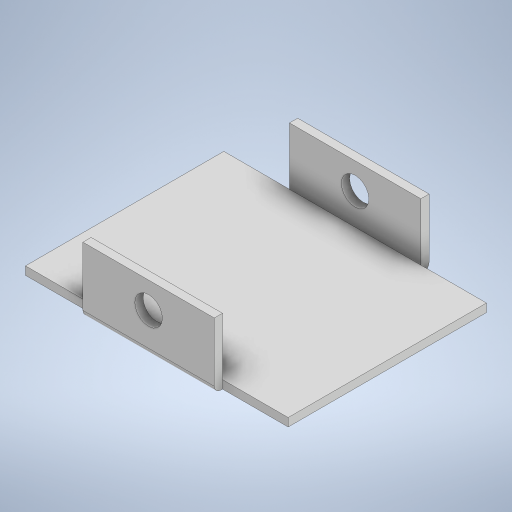
# Autodesk Inventor part: L1 Gearbox Cover Top
Saved by Autodesk Inventor 2024 (Build 280153000, 153)
## iProperties
Created: 2023-09-27
Part Number: L1 Gearbox Cover Top
Material: Generic
Document SubType Name: Modeling
Designer: lando
Density: 1 g/cm^3
Appearance: Default
Author: lando
Autodesk Inventor part; units mm, degrees
ref_plane "YZ Plane" through (0, 0, 0) normal (1, 0, 0) x (0, 1, 0)
ref_plane "XZ Plane" through (0, 0, 0) normal (0, 1, 0) x (-1, 0, 0)
ref_plane "XY Plane" through (0, 0, 0) normal (0, 0, 1) x (1, 0, 0)
sketch "Sketch1" plane through (0, 0, 0) normal (0, 1, 0) x (-1, 0, 0)
  line L0 (0, 0) -> (50.8, 0)
  line L1 (50.8, 0) -> (50.8, -38.354)
  line L2 (50.8, -38.354) -> (0, -38.354)
  line L3 (0, -38.354) -> (0, 0)
  dimension "d0" = 50.8
  dimension "d1" = 38.354
  constraints: 8 end point, 2 parallel, 1 horizontal, 1 perpendicular
  measures "d0" distance of L1.end L2.end
  measures "d1" distance of L0.end L1.end
extrude "Extrusion1" add sketch "Sketch1" along normal blind 1.5875
sketch "Sketch2" plane through (-50.8, 0, 0) normal (0, 0, 1) x (1, 0, 0)
  line L0 (50.8, 0) -> (0, 0) projected
  line L1 (50.8, 0) -> (38.1, 0)
  line L2 (38.1, 0) -> (12.7, 0)
  line L3 (12.7, 0) -> (12.7, 12.7)
  line L4 (12.7, 12.7) -> (38.1, 12.7)
  line L5 (38.1, 12.7) -> (38.1, 0)
  line L6 (50.8, 1.5875) -> (0, 1.5875) projected
  dimension "d4" = 12.7
  dimension "d5" = 25.4
  dimension "d6" = 12.7
  constraints: 10 end point, 3 perpendicular, 2 point on line
  measures "d4" distance of L0.start L1.end
  measures "d5" distance of L1.end L2.end
  measures "d6" distance of L2.end L3.end
extrude "Extrusion2" add sketch "Sketch2" along normal blind 1.5875
sketch "Sketch3" plane through (0, 0, -38.354) normal (0, 0, -1) x (-1, 0, 0)
  line L0 (0, 0) -> (0, 1.5875) projected
  line L1 (12.7, 0) -> (0, 0) projected
  line L2 (0, 0) -> (12.7, 0)
  line L3 (12.7, 0) -> (38.1, 0)
  line L4 (38.1, 0) -> (38.1, 12.7)
  line L5 (38.1, 12.7) -> (12.7, 12.7)
  line L6 (12.7, 12.7) -> (12.7, 0)
  dimension "d9" = 12.7
  dimension "d10" = 25.4
  dimension "d11" = 12.7
  dimension "d12" = 25.4
  constraints: 10 end point, 2 perpendicular, 1 collinear, 1 point on line
  measures "d9" distance of L0.start L1.start
  measures "d10" distance of L1.start L3.end
  measures "d11" distance of L3.end L4.end
  measures "d12" distance of L4.end L5.end
extrude "Extrusion3" add sketch "Sketch3" along normal blind 1.5875
sketch "Sketch4" plane through (0, 0, -39.9415) normal (0, 0, -1) x (-1, 0, 0)
  circle A0 centre (25.4, 7.62) radius 2.667
  line L0 (38.1, 0) -> (38.1, 12.7) projected
  line L1 (38.1, 12.7) -> (12.7, 12.7) projected
  point P0 (0, 0)
  dimension "d15" = 12.7
  dimension "d16" = 5.08
  dimension "d17" = 5.334
  constraints: 1 centre point
  measures "d15" distance from line of L0 A0.centre
  measures "d16" distance from line of L1 A0.centre
  measures "d17" diameter of A0
extrude "Extrusion4" cut sketch "Sketch4" against normal blind 50.8
fillet "Fillet1" radius 1.27 2 edges at (-25.4, 0, -39.9415) (-25.4, 0, 1.5875)
body "Solid1"
